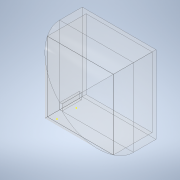
# Autodesk Inventor part: Deckel
Saved by Autodesk Inventor 2020 (Build 240168000, 168)
## iProperties
Created: 2021-06-29
Part Number: Deckel
Material: PMMA-Kunststoff
Document SubType Name: Modeling
Designer: Julian Uhl
Density: 1.188 g/cm^3
Appearance: Polycarbonat - klar
Author: Julian Uhl
Autodesk Inventor part; units mm, degrees
ref_plane "YZ Plane" through (0, 0, 0) normal (1, 0, 0) x (0, 1, 0)
ref_plane "XZ Plane" through (0, 0, 0) normal (0, 1, 0) x (-1, 0, 0)
ref_plane "XY Plane" through (0, 0, 0) normal (0, 0, 1) x (1, 0, 0)
sketch "Skizze1" plane through (0, 0, 0) normal (0, 0, 1) x (1, 0, 0)
  line L0 (-123.0333, 0) -> (142.9667, 0) projected
  line L1 (0, -107.5057) -> (0, 172.4943) projected
  line L2 (-75.0333, 122.4943) -> (94.9667, 122.4943)
  line L3 (94.9667, 122.4943) -> (94.9667, -57.5057)
  line L4 (94.9667, -57.5057) -> (-75.0333, -57.5057)
  line L5 (-75.0333, -57.5057) -> (-75.0333, 122.4943)
  line L6 (-85.0333, 132.4943) -> (104.9667, 132.4943)
  line L7 (104.9667, 132.4943) -> (104.9667, -67.5057)
  line L8 (104.9667, -67.5057) -> (-85.0333, -67.5057)
  line L9 (-85.0333, -67.5057) -> (-85.0333, 132.4943)
  point P0 (0, 0)
  dimension "d0" = 170
  dimension "d1" = 180
  dimension "d2" = 10
  dimension "d3" = 10
  dimension "d4" = 10
  dimension "d5" = 10
  constraints: 16 end point, 4 parallel, 2 horizontal, 2 perpendicular
  measures "d0" distance between parallel lines of L3 L5
  measures "d1" distance between parallel lines of L4 L2
  measures "d2" distance between parallel lines of L6 L2
  measures "d3" distance between parallel lines of L7 L3
  measures "d4" distance between parallel lines of L8 L4
  measures "d5" distance between parallel lines of L9 L5
extrude "Extrusion1" add sketch "Skizze1" along normal blind 100 contours L9 L6 L1 L2 L5 L0 | L0 L5 L4 L1 L8 L9 | L1 L4 L3 L0 L7 L8 | L6 L7 L0 L3 L2 L1
sketch "Skizze2" plane through (0, 0, 100) normal (0, 0, 1) x (1, 0, 0)
  point P0 (0, 0)
sketch "Skizze3" plane through (0, 0, 100) normal (0, 0, 1) x (1, 0, 0)
  line L0 (-85.0333, 132.4943) -> (-85.0333, -67.5057) projected
  line L1 (-85.0333, 132.4943) -> (104.9667, 132.4943)
  line L2 (104.9667, 132.4943) -> (104.9667, -67.5057)
  line L3 (104.9667, -67.5057) -> (-85.0333, -67.5057)
  line L4 (-85.0333, -67.5057) -> (-85.0333, 132.4943)
  point P0 (0, 0)
  constraints: 8 end point, 2 parallel, 1 horizontal, 1 perpendicular
extrude "Extrusion2" add sketch "Skizze3" along normal blind 50
fillet "Rundung1" radius 92 4 edges at (-85.0333, 32.4943, 150) (9.9667, 132.4943, 150) (9.9667, -67.5057, 150) (104.9667, 32.4943, 150)
sketch "Skizze4" plane through (0, 0, 150) normal (0, 0, 1) x (1, 0, 0)
  point P0 (0, 0)
sketch "Skizze5" plane through (0, 0, 150) normal (0, 0, 1) x (1, 0, 0)
  line L0 (6.9667, 24.4943) -> (6.9667, 40.4943) projected
  line L1 (94.8203, -57.3593) -> (12.9667, 24.4943) projected
  line L2 (6.9667, 40.4943) -> (12.9667, 40.4943)
  line L3 (12.9667, 40.4943) -> (12.9667, 24.4943)
  line L4 (12.9667, 24.4943) -> (6.9667, 24.4943)
  line L5 (6.9667, 24.4943) -> (6.9667, 40.4943)
  point P0 (0, 0)
  constraints: 8 end point, 2 parallel, 1 horizontal, 1 perpendicular
extrude "Extrusion3" cut sketch "Skizze5" against normal blind 50
